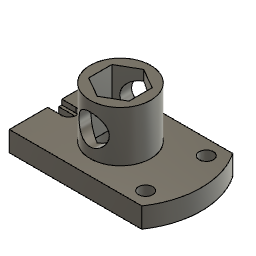
drawing_19 v1 (Autodesk Fusion 360 design; units mm, degrees)
Autodesk Fusion 360 part; units mm, degrees
note: some values were not read from the file. Set by a fixed rule: which sketch regions a step uses.
sketch "Sketch1" plane through (0, 0, 0) normal (0, 1, 0) x (1, 0, 0)
  line L0 (58.6438, 45) -> (-72.5, 45)
  line L1 (-72.5, 45) -> (-72.5, -45)
  line L2 (-72.5, -45) -> (58.6438, -45)
  line L3 (62.4739, 38.7769) -> (-72.5, -45) construction
  line L4 (-72.5, 45) -> (62.4739, -38.7769) construction
  line L5 (-72.5, 0) -> (-7.5, 0)
  arc A0 (58.6438, -45) -> (58.6438, 45) centre (-7.5, 0) ccw
  circle A1 centre (-7.5, 0) radius 23
  dimension "d2" = 90
  dimension "d3" = 65
  dimension "d4" = 160
  dimension "d7" = 46
  constraint horizontal L0
  constraint perpendicular L0 L1
  constraint parallel L0 L2
  constraint coincident L3 origin
  constraint coincident L4 origin
  constraint midpoint L1 L5.start
  constraint perpendicular L1 L5
  constraint coincident L5.end A0.centre
  constraint coincident A0 L4.end
  constraint coincident A0 L3.start
  constraint concentric A0 A1
  measures "d2" distance of L0.end L1.end
  measures "d3" distance of L5.start L5.end
  measures "d4" diameter of A0
  measures "d7" diameter of A1
extrude "Extrude2" add sketch "Sketch1" along normal blind 15 contours A1 makes body 1
extrude "Extrude1" add sketch "Sketch1" along normal blind 20 separate body contours L0 L1 L2 A0 | A1 makes body 2
combine "Combine1" operation cut target body 2 tool bodies 1
sketch "Sketch2" plane through (0, 20, 0) normal (0, 1, 0) x (-1, 0, 0)
  arc A0 (-58.6438, 45) -> (-58.6438, -45) centre (7.5, 0) ccw
  line L0 (-58.6438, -45) -> (72.5, -45)
  line L1 (72.5, -45) -> (72.5, 45)
  line L2 (72.5, 45) -> (-58.6438, 45)
  circle A1 centre (7.5, 0) radius 23
  circle A2 centre (7.5, 0) radius 30
  dimension "d10" = 60
  constraint concentric A1 A2
  measures "d10" diameter of A2
extrude "Extrude3" add sketch "Sketch2" along normal blind 50 contours A1 | A2 bodies 2
sketch "Sketch3" plane through (0, 70, 0) normal (0, 1, 0) x (-1, 0, 0)
  circle A0 centre (7.5, 0) radius 30
  line L0 (7.5, -23) -> (27.4186, -11.5)
  line L1 (27.4186, -11.5) -> (27.4186, 11.5)
  line L2 (27.4186, 11.5) -> (7.5, 23)
  line L3 (7.5, 23) -> (-12.4186, 11.5)
  line L4 (-12.4186, 11.5) -> (-12.4186, -11.5)
  line L5 (-12.4186, -11.5) -> (7.5, -23)
  point P0 (7.5, 0)
  dimension "d13" = 23
  constraint coincident P0 A0.centre
  measures "d13" distance of L0.start P0
extrude "Extrude4" cut sketch "Sketch3" against normal blind 55 contours L0 L1 L2 L3 L4 L5 bodies 2
ref_plane "WorkPlane1" through (-6.9281, 10, 45) normal (0, 0, 1) x (1, 0, 0)
sketch "Sketch4" plane through (-6.9281, 10, 45) normal (0, 0, 1) x (1, 0, 0)
  line L0 (29.4281, 60) -> (-30.5719, 60)
  line L1 (-30.5719, 10) -> (29.4281, 10)
  line L2 (-0.5719, 60) -> (-0.5719, 35)
  circle A0 centre (-0.5719, 35) radius 15
  dimension "d17" = 25
  dimension "d18" = 30
  constraint midpoint L0 L2.start
  constraint perpendicular L0 L2
  constraint coincident L2.end A0.centre
  measures "d17" distance of L2.start L2.end
  measures "d18" diameter of A0
extrude "Extrude5" cut sketch "Sketch4" against normal blind 135 bodies 2
sketch "Sketch5" plane through (0, 20, 0) normal (0, 1, 0) x (-1, 0, 0)
  circle A0 centre (7.5, 0) radius 30
  arc A1 (-58.6438, 45) -> (-58.6438, -45) centre (7.5, 0) ccw
  line L0 (-58.6438, -45) -> (72.5, -45)
  line L1 (72.5, -45) -> (72.5, 45)
  line L2 (72.5, 45) -> (-58.6438, 45)
  line L3 (-47.5, -30) -> (62.5, -30)
  line L4 (62.5, -30) -> (62.5, 30)
  line L5 (62.5, 30) -> (-47.5, 30)
  line L6 (-47.5, 30) -> (-47.5, -30)
  line L7 (-47.5, -30) -> (62.5, 30) construction
  line L8 (62.5, -30) -> (-47.5, 30) construction
  line L9 (72.5, -45) -> (58.5, -45)
  line L10 (58.5, -45) -> (58.5, -30)
  line L11 (58.5, -30) -> (72.5, -30)
  line L12 (72.5, -30) -> (72.5, -45)
  circle A2 centre (-47.5, -30) radius 7
  circle A3 centre (-47.5, 30) radius 7
  circle A4 centre (58.5, -30) radius 8
  point P0 (7.5, 0)
  dimension "d21" = 110
  dimension "d22" = 60
  dimension "d23" = 14
  dimension "d24" = 15
  dimension "d25" = 14
  dimension "d26" = 14
  dimension "d27" = 16
  constraint horizontal L3
  constraint perpendicular L3 L4
  constraint parallel L3 L5
  constraint parallel L4 L6
  constraint coincident L7 P0
  constraint coincident L8 P0
  constraint coincident P0 A0.centre
  constraint horizontal L9
  constraint vertical L10
  constraint horizontal L11
  constraint vertical L12
  constraint coincident L0.end L1.start
  constraint coincident L3.start L6.end
  constraint coincident L5.end L6.start
  constraint coincident L10.end L11.start
  measures "d21" distance of L4.end L5.end
  measures "d22" distance of L3.end L4.end
  measures "d23" distance of L0.end L9.end
  measures "d24" distance of L0.end L11.end
  measures "d25" diameter of A2
  measures "d26" diameter of A3
  measures "d27" diameter of A4
extrude "Extrude6" cut sketch "Sketch5" against normal blind 20 contours L5 L6 A3 | L5 L6 A3 | L3 L6 A2 | L3 L6 A2 | L3 L4 L11 A4 | L3 L10 A4 | L4 L11 A4 | L3 L10 L11 A4 bodies 2
sketch "Sketch6" plane through (0, 20, 0) normal (0, 1, 0) x (-1, 0, 0)
  circle A0 centre (-47.5, 30) radius 7
  circle A1 centre (-47.5, -30) radius 7
  circle A2 centre (58.5, -30) radius 8
  circle A3 centre (7.5, 0) radius 30
  arc A4 (-58.6438, 45) -> (-58.6438, -45) centre (7.5, 0) ccw
  line L0 (-58.6438, -45) -> (72.5, -45)
  line L1 (72.5, -45) -> (72.5, 45)
  line L2 (72.5, 45) -> (-58.6438, 45)
  line L3 (58.5, -30) -> (58.5, 30) construction
  line L4 (72.5, 0) -> (58.5, 0) construction
  line L5 (58.5, -7) -> (79, -7)
  arc A5 (79, -7) -> (79, 7) centre (79, 0) ccw
  line L6 (79, 7) -> (58.5, 7)
  arc A6 (58.5, 7) -> (58.5, -7) centre (58.5, 0) ccw
  line L7 (58.5, 0) -> (79, 0) construction
  dimension "d30" = 14
  constraint coincident A2.centre L3.start
  constraint vertical L3
  constraint midpoint L1 L4.start
  constraint midpoint L3 L4.end
  constraint tangent L5 A5
  constraint tangent A5 L6
  constraint parallel L5 L6
  constraint tangent L6 A6
  constraint tangent L5 A6
  constraint perpendicular L1 L7
  constraint coincident L4.end A6.centre
  measures "d30" diameter of A5
extrude "Extrude7" cut sketch "Sketch6" against normal blind 5 contours L1 L5 L6 A6 bodies 2
sketch "Sketch7" plane through (0, 15, 0) normal (0, 1, 0) x (-1, 0, 0)
  arc A0 (58.5, 7) -> (58.5, -7) centre (58.5, 0) ccw
  line L0 (58.5, -7) -> (72.5, -7)
  line L1 (72.5, -7) -> (72.5, 7)
  line L2 (72.5, 7) -> (58.5, 7)
  line L3 (58.5, -4) -> (88, -4)
  arc A1 (88, -4) -> (88, 4) centre (88, 0) ccw
  line L4 (88, 4) -> (58.5, 4)
  arc A2 (58.5, 4) -> (58.5, -4) centre (58.5, 0) ccw
  line L5 (58.5, 0) -> (88, 0) construction
  dimension "d33" = 8
  constraint tangent L3 A1
  constraint tangent A1 L4
  constraint parallel L3 L4
  constraint tangent L4 A2
  constraint tangent L3 A2
  constraint horizontal L5
  constraint coincident A0.centre A2.centre
  measures "d33" diameter of A1
extrude "Extrude8" cut sketch "Sketch7" against normal blind 20 contours L1 L3 L4 A2 bodies 2
equation "d4 = ( 80 * 2 ) * 1 mm"
equation "d11 = 70 mm - 20 mm"
equation "d13 = ( 46 / 2 ) * 1 mm"
equation "d21 = ( 55 * 2 ) * 1 mm"
